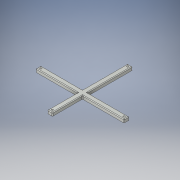
# Autodesk Inventor part: BatteryCrossStrap
Saved by Autodesk Inventor 2016 (Build 200138000, 138)
## iProperties
Created: 2015-09-14
Part Number: BatteryCrossStrap
Material: Generic
Document SubType Name: Modeling
Designer: lachesis
Density: 1 g/cm^3
Appearance: Default
Author: lachesis
Autodesk Inventor part; units mm, degrees
ref_plane "YZ Plane" through (0, 0, 0) normal (1, 0, 0) x (0, 1, 0)
ref_plane "XZ Plane" through (0, 0, 0) normal (0, 1, 0) x (-1, 0, 0)
ref_plane "XY Plane" through (0, 0, 0) normal (0, 0, 1) x (1, 0, 0)
sketch "Sketch1" plane through (0, 0, 0) normal (0, 1, 0) x (-1, 0, 0)
  line L0 (84.709, 4.7625) -> (-84.709, 4.7625)
  line L1 (-84.709, 4.7625) -> (-84.709, -4.7625)
  line L2 (-84.709, -4.7625) -> (84.709, -4.7625)
  line L3 (84.709, -4.7625) -> (84.709, 4.7625)
  line L4 (4.7625, 62.5475) -> (-4.7625, 62.5475)
  line L5 (-4.7625, 62.5475) -> (-4.7625, -91.4781)
  line L6 (-4.7625, -91.4781) -> (4.7625, -91.4781)
  line L7 (4.7625, -91.4781) -> (4.7625, 62.5475)
  point P0 (0, 0)
  point P1 (0, -4.7625)
  point P2 (84.709, 0)
  point P3 (4.7625, -14.4653)
  point P4 (0, 62.5475)
  dimension "d0" = 9.525
  dimension "d1" = 169.418
  dimension "d2" = 154.0256
  dimension "d6" = 57.785
  constraints: 16 end point, 4 midpoint, 4 parallel, 3 perpendicular, 2 horizontal, 2 vertical alignment, 1 horizontal alignment
  measures "d0" distance of L2.end L0.start
  measures "d1" distance of L1.end L2.end
  measures "d2" distance of L6.end L4.start
  measures "d6" distance between parallel lines of L4 L0
extrude "Extrusion1" add sketch "Sketch1" along normal blind 6.35
sketch "Sketch2" plane through (0, 6.35, 0) normal (0, 1, 0) x (1, 0, 0)
  line L0 (4.7625, 91.4781) -> (-4.7625, 91.4781) projected
  line L1 (84.709, -4.7625) -> (84.709, 4.7625) projected
  line L2 (-4.7625, -62.5475) -> (4.7625, -62.5475) projected
  line L3 (-84.709, 4.7625) -> (-84.709, -4.7625) projected
  point P0 (0, 0)
  point P1 (0, 86.7791)
  point P2 (0, -57.8485)
  point P3 (-80.01, 0)
  point P4 (80.01, 0)
  dimension "d7" = 4.699
  dimension "d8" = 4.699
  dimension "d9" = 4.699
  dimension "d10" = 4.699
  constraints: 2 horizontal alignment, 2 vertical alignment
  measures "d7" distance from line of L0 point (0, 86.779)
  measures "d8" distance from line of L1 point (80.01, 0)
  measures "d9" distance from line of L2 point (0, -57.849)
  measures "d10" distance from line of L3 point (-80.01, 0)
hole "Hole1" at (0, 6.35, -86.7791) at (0, 6.35, 57.8485) at (-80.01, 6.35, 0) at (80.01, 6.35, 0) direction (0, -1, 0) diameter 3.302 end through all
fillet "Fillet1" radius 1.27 20 edges at (-44.7358, 6.35, 4.7625) (4.7625, 6.35, 33.655) (-4.7625, 6.35, 33.655) (44.7357, 6.35, 4.7625) (4.7625, 6.35, -48.1203) (-4.7625, 6.35, -48.1203) (-44.7357, 6.35, -4.7625) (44.7358, 6.35, -4.7625) (84.709, 3.175, 4.7625) (84.709, 3.175, -4.7625) (84.709, 6.35, 0) (4.7625, 3.175, 62.5475) (0, 6.35, 62.5475) (-4.7625, 3.175, 62.5475) (-84.709, 3.175, 4.7625) (-84.709, 6.35, 0) (4.7625, 3.175, -91.4781) (0, 6.35, -91.4781) (-4.7625, 3.175, -91.4781) (-84.709, 3.175, -4.7625)
fillet "Fillet2" radius 1.27 8 edges at (4.3905, 5.978, 4.3905) (4.7625, 2.54, 4.7625) (4.3905, 5.978, -4.3905) (4.7625, 2.54, -4.7625) (-4.3905, 5.978, -4.3905) (-4.7625, 2.54, -4.7625) (-4.3905, 5.978, 4.3905) (-4.7625, 2.54, 4.7625)
equation "\"d8\" = d7"
equation "\"d9\" = d7"
equation "\"d10\" = d7"
body "Solid1"
